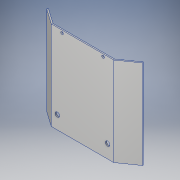
# Autodesk Inventor part: solar sheild
Saved by Autodesk Inventor 2017 (Build 210142000, 142)
## iProperties
Created: 2017-03-06
Part Number: solar sheild
Material: Aluminum 6061
Document SubType Name: Modeling
Designer: qupec
Density: 2.7 g/cm^3
Appearance: Aluminum - Flat
Author: qupec
Autodesk Inventor part; units mm, degrees
ref_plane "YZ Plane" through (0, 0, 0) normal (1, 0, 0) x (0, 1, 0)
ref_plane "XZ Plane" through (0, 0, 0) normal (0, 1, 0) x (-1, 0, 0)
ref_plane "XY Plane" through (0, 0, 0) normal (0, 0, 1) x (1, 0, 0)
sketch "Sketch1" plane through (0, 0, 0) normal (0, 1, 0) x (-1, 0, 0)
  line L0 (-38.6259, 0.7937) -> (38.6259, 0.7937)
  line L1 (-38.1254, -0.7938) -> (-38.6259, 0.7937) construction
  line L2 (-38.6259, 0.7937) -> (-59.8424, -14.0622)
  line L3 (-59.8424, -14.0622) -> (-58.9319, -15.3626)
  line L4 (-58.9319, -15.3626) -> (-38.1254, -0.7938)
  line L5 (-38.1254, -0.7938) -> (38.1254, -0.7938)
  line L6 (38.1254, -0.7938) -> (56.6432, -13.76)
  line L7 (56.6432, -13.76) -> (57.5537, -12.4596)
  line L8 (57.5537, -12.4596) -> (38.6259, 0.7937)
  point P0 (0, 0)
  dimension "d75" = 1.5875
  dimension "d76" = 1.5875
  dimension "d77" = 1.5875
  dimension "d78" = 145
  dimension "d79" = 76.2508
  dimension "d80" = 38.1254
  dimension "d81" = 0.7937
  dimension "d82" = 145
  dimension "d83" = 22.606
  dimension "d84" = 25.4
  constraints: 18 end point, 3 perpendicular, 2 horizontal
  measures "d75" distance between parallel lines of L4 L2
  measures "d76" distance between parallel lines of L6 L8
  measures "d77" distance between parallel lines of L5 L0
  measures "d78" angle of L5 L4
  measures "d79" distance of L1.start L5.end
  measures "d80" horizontal distance of point (0, 0) L1.start
  measures "d81" distance from line of point (0, 0) L0
  measures "d82" angle of L5 L6
  measures "d83" distance from line of L5.end L7
  measures "d84" distance from line of L1.start L3
extrude "Extrusion1" add sketch "Sketch1" along normal blind 109.855
sketch "Sketch2" plane through (38.1254, 0, -0.7938) normal (0, 0, -1) x (-1, 0, 0)
  circle A0 centre (7.0104, 16.51) radius 2.794
  circle A1 centre (69.2404, 16.51) radius 2.794
  line L0 (76.7513, 0) -> (-0.5005, 0)
  line L1 (38.1254, 97.155) -> (38.1254, 0) construction
  line L2 (0, 0) -> (0, 109.855) projected
  line L3 (76.2508, 0) -> (76.2508, 109.855) projected
  point P0 (33.1273, 0)
  dimension "d21" = 5.588
  dimension "d22" = 5.588
  dimension "d23" = 62.23
  dimension "d28" = 16.51
  dimension "d29" = 16.51
  dimension "d91" = 31.115
  dimension "d101" = 76.2508
  dimension "d102" = 38.1254
  constraints: 4 end point, 2 centre point, 1 midpoint
  measures "d21" diameter of A0
  measures "d22" diameter of A1
  measures "d23" distance of A1.centre A0.centre
  measures "d28" distance from line of L0 A0.centre
  measures "d29" distance from line of L0 A1.centre
  measures "d91" distance from line of L1 A0.centre
  measures "d101" distance between parallel lines of L3 L2
  measures "d102" distance between parallel lines of L1 L2
extrude "Extrusion2" cut sketch "Sketch2" against normal through all
sketch "Sketch3" plane through (38.1254, 0, -0.7938) normal (0, 0, -1) x (-1, 0, 0)
  line L0 (38.1254, 97.0628) -> (38.1254, 73.759) construction
  line L1 (76.2508, 0) -> (76.2508, 109.855) construction
  line L2 (0, 0) -> (0, 109.855) construction
  line L3 (76.7513, 109.855) -> (-0.5005, 109.855) construction
  point P0 (38.1254, 0)
  point P1 (12.7254, 106.68)
  point P2 (63.5254, 106.68)
  dimension "d85" = 76.2508
  dimension "d86" = 38.1254
  dimension "d87" = 25.4
  dimension "d88" = 3.175
  dimension "d93" = 50.8
  constraints: 2 end point, 1 vertical
  measures "d85" distance between parallel lines of L1 L2
  measures "d86" distance between parallel lines of L0 L2
  measures "d87" distance from line of L0 point (12.725, 106.68)
  measures "d88" distance from line of L3 point (12.725, 106.68)
  measures "d93" distance of point (63.525, 106.68) point (12.725, 106.68)
hole "Hole1" at (25.4, 106.68, -0.7938) at (-25.4, 106.68, -0.7938) direction (0, 0, 1) diameter 3.2004 depth 25.4 tip angle 118
equation "\"d75\" = d77"
equation "\"d76\" = d77"
equation "\"d80\" = 0.5 * d79"
equation "\"d81\" = 0.5 * d77"
equation "\"d22\" = d21"
equation "\"d29\" = d28"
equation "\"d91\" = 0.5 * d23"
equation "\"d102\" = 0.5 * d101"
equation "\"d86\" = 0.5 * d85"
equation "\"d87\" = 0.5 * d93"
body "Solid1"
